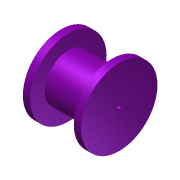
# Autodesk Inventor part: Spool
Saved by Autodesk Inventor 2011 (Build 150239000, 239)
## iProperties
Created: 2014-09-16
Part Number: Spool
Document SubType Name: Modeling
Designer: Family Room
Density: 1 g/cm^3
Author: Family Room
Autodesk Inventor part; units mm, degrees
ref_plane "YZ Plane" through (0, 0, 0) normal (1, 0, 0) x (0, 1, 0)
ref_plane "XZ Plane" through (0, 0, 0) normal (0, 1, 0) x (-1, 0, 0)
ref_plane "XY Plane" through (0, 0, 0) normal (0, 0, 1) x (1, 0, 0)
sketch "Sketch1" plane through (0, 0, 0) normal (0, 0, 1) x (1, 0, 0)
  line L0 (-19.05, 25.0245) -> (19.05, 25.0245)
  line L1 (19.05, 25.0245) -> (19.05, 44.0745)
  line L2 (19.05, 44.0745) -> (-19.05, 44.0745)
  line L3 (-19.05, 44.0745) -> (-19.05, 25.0245)
  line L4 (19.05, 56.7745) -> (25.4, 56.7745)
  line L5 (25.4, 56.7745) -> (25.4, 25.0245)
  line L6 (25.4, 25.0245) -> (19.05, 25.0245)
  line L7 (19.05, 25.0245) -> (19.05, 56.7745)
  line L8 (-19.05, 56.7745) -> (-25.4, 56.7745)
  line L9 (-25.4, 56.7745) -> (-25.4, 25.0245)
  line L10 (-25.4, 25.0245) -> (-19.05, 25.0245)
  line L11 (-19.05, 25.0245) -> (-19.05, 56.7745)
  line L12 (-27.7097, 23.437) -> (29.609, 23.437)
  point P0 (0, 0)
  dimension "d0" = 38.1
  dimension "d1" = 19.05
  dimension "d2" = 6.35
  dimension "d3" = 31.75
  dimension "d4" = 12.7
  dimension "d5" = 6.35
  dimension "d6" = 1.5875
  dimension "d8" = 31.75
  constraints: 26 end point, 6 parallel, 4 perpendicular, 3 horizontal, 1 collinear
  measures "d0" distance of L2.end L1.end
  measures "d1" distance of L1.end L0.end
  measures "d2" distance of L5.end L6.end
  measures "d3" distance of L4.end L5.end
  measures "d4" distance between parallel lines of L2 L4
  measures "d5" distance of L10.end L9.end
  measures "d6" distance between parallel lines of L0 L12
  measures "d8" distance of L8.end L9.end
revolve "Revolution1" add sketch "Sketch1" angle 360 about axis through (-27.7097, 23.437, 0) along (1, 0, 0)
body "Solid1"
